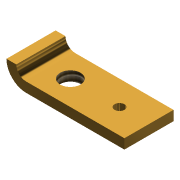
# Autodesk Inventor part: contact
Saved by Autodesk Inventor 2022 (Build 260148000, 148)
## iProperties
Shininess: 64.0
Length Units: 11272
Angle Units: 11279
Time Units: 11290
Mass Units: 11286
Length Display Precision: 3
Angle Display Precision: 2
Created: 2002-05-01
Part Number: contact
Material: Brass, Soft Yellow
Document SubType Name: Modeling
Designer: Administrator
Density: 8.47 g/cm^3
Appearance: Brass - Satin
Density: 8.47
Volumn: 0.11798191640455558
Area: 2.5739262989165304
PropertySet Name: Model Information
Control State: 0
Master: False
Checked Out: False
Author: Administrator
Autodesk Inventor part; units mm, degrees
ref_plane "YZ Plane" through (0, 0, 0) normal (1, 0, 0) x (0, 1, 0)
ref_plane "XZ Plane" through (0, 0, 0) normal (0, 1, 0) x (-1, 0, 0)
ref_plane "XY Plane" through (0, 0, 0) normal (0, 0, 1) x (1, 0, 0)
sketch "Sketch1" plane through (0, 0, 0) normal (0, 0, 1) x (1, 0, 0)
  line L0 (-37.1688, 9.374) -> (-37.1688, 9.374)
  line L1 (-34.6288, 6.834) -> (-21.9288, 6.834)
  line L2 (-21.9288, 6.834) -> (-21.9288, 8.104)
  line L3 (-21.9288, 8.104) -> (-34.6288, 8.104)
  line L4 (-35.8988, 9.374) -> (-35.8988, 9.374)
  line L5 (-35.8988, 9.374) -> (-37.1688, 9.374)
  arc A0 (-35.8988, 9.374) -> (-34.6288, 8.104) centre (-34.6288, 9.374) ccw
  arc A1 (-37.1688, 9.374) -> (-34.6288, 6.834) centre (-34.6288, 9.374) ccw
  dimension "d0" = 1.27
  dimension "d1" = 1.27
  dimension "d2" = 2.54
  dimension "d3" = 1.27
  dimension "d4" = 15.24
  dimension "d5" = 2.54
  constraints: 12 end point, 4 parallel, 4 point on circle, 4 tangent, 2 centre point, 1 perpendicular, 1 vertical
  measures "d0" distance of L1.end L2.end
  measures "d1" radius of A0
  measures "d2" radius of A1
  measures "d3" distance of L4.end L0.start
  measures "d4" distance from line of L1.end L0
  measures "d5" distance from line of L0.start L1
extrude "Extrusion1" add sketch "Sketch1" along normal blind 6.35
sketch "Sketch2" plane through (-34.6288, 8.104, 0) normal (0, 1, 0) x (1, 0, 0)
  line L0 (0, -6.35) -> (12.7, -6.35) projected
  line L1 (0, 0) -> (12.7, 0) projected
  circle A0 centre (2.54, -3.175) radius 3.175 construction
  dimension "d8" = 10.16
  constraints: 2 tangent, 1 centre point, 1 coincident
  measures "d8" horizontal distance of L0.end A0.centre
hole "Hole1" at (-32.0888, 8.104, 3.175) at (-32.0888, 8.104, 3.175) direction (0, -1, 0) diameter 2.6416 end through all thread size "6-32 UNC" class "2B" standard "ANSI Unified Screw Threads"
sketch "Sketch3" plane through (-34.6288, 8.104, 0) normal (0, 1, 0) x (1, 0, 0)
  circle A0 centre (2.54, -3.175) radius 1.3208 projected
  point P0 (8.89, -3.175)
  dimension "d16" = 6.35
  constraints: 1 horizontal alignment
  measures "d16" distance of point (8.89, -3.175) A0.centre
hole "Hole2" at (-25.7388, 8.104, 3.175) direction (0, -1, 0) diameter 1.27 end through all
body "Solid1"
